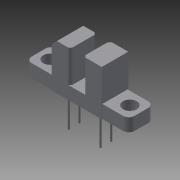
# Autodesk Inventor part: Capteur optique
Saved by Autodesk Inventor 2015 SP1 (Build 190203100, 203)
## iProperties
Created: 2015-05-01
Part Number: Capteur optique
Material: Générique
Document SubType Name: Modeling
Designer: Cyril
Density: 1 g/cm^3
Appearance: Par défaut
Author: Cyril
Autodesk Inventor part; units mm, degrees
ref_plane "YZ Plane" through (0, 0, 0) normal (1, 0, 0) x (0, 1, 0)
ref_plane "XZ Plane" through (0, 0, 0) normal (0, 1, 0) x (-1, 0, 0)
ref_plane "XY Plane" through (0, 0, 0) normal (0, 0, 1) x (1, 0, 0)
sketch "Sketch1" plane through (0, 0, 0) normal (0, 1, 0) x (-1, 0, 0)
  line L0 (-1.55, 2.6) -> (-5.95, 2.6)
  line L1 (-5.95, 2.6) -> (-5.95, -8.2)
  line L2 (-5.95, -8.2) -> (5.95, -8.2)
  line L3 (5.95, -8.2) -> (5.95, 1.4)
  line L4 (5.95, 1.4) -> (4.75, 2.6)
  line L5 (4.75, 2.6) -> (1.55, 2.6)
  line L6 (1.55, 2.6) -> (1.55, -5.1)
  line L7 (1.55, -5.1) -> (-1.55, -5.1)
  line L8 (-1.55, -5.1) -> (-1.55, 2.6)
  line L9 (0, -10.36) -> (0, 4.76) projected
  point P0 (0, 0)
  dimension "d0" = 11.9
  dimension "d1" = 10.8
  dimension "d2" = 2.6
  dimension "d3" = 3.1
  dimension "d4" = 3.1
  dimension "d5" = 135
  dimension "d6" = 1.2
  constraints: 18 end point, 6 perpendicular, 2 point on line, 1 horizontal, 2 other
  measures "d0" distance of L1.end L2.end
  measures "d1" distance of L0.end L1.end
  measures "d2" distance from line of point (0, 0) L0
  measures "d3" distance between parallel lines of L8 L6
  measures "d4" distance between parallel lines of L7 L2
  measures "d5" angle of L5 L4
  measures "d6" distance from line of L4.end L3
extrude "Extrusion1" add sketch "Sketch1" along normal mid plane 6.3
sketch "Sketch2" plane through (5.95, -3.15, -8.2) normal (1, 0, 0) x (0, 0, -1)
  line L0 (0, 0.15) -> (-3.1, 0.15)
  line L1 (-3.1, 0.15) -> (-3.1, 6.15)
  line L2 (-3.1, 6.15) -> (0, 6.15)
  line L3 (0, 6.15) -> (0, 0.15)
  line L4 (2.16, 3.15) -> (-12.96, 3.15) projected
  point P0 (-8.2, 3.15)
  point P1 (0, 0)
  dimension "d12" = 6
  dimension "d13" = 3.1
  constraints: 8 end point, 2 parallel, 1 horizontal, 1 perpendicular, 1 point on line, 1 other
  measures "d12" distance of L0.end L1.end
  measures "d13" distance of L1.end L2.end
extrude "Extrusion2" add sketch "Sketch2" along normal blind 6.3
fillet "Fillet1" radius 1.35 2 edges at (12.25, -3, -6.65) (12.25, 3, -6.65)
sketch "Sketch3" plane through (5.95, -3, -5.1) normal (0, 0, 1) x (1, 0, 0)
  circle A0 centre (3.55, 3) radius 1.65
  line L0 (0, -0.15) -> (0, 6.15) projected
  line L1 (-15.54, 3) -> (9.94, 3) projected
  point P0 (-5.95, 3)
  dimension "d15" = 3.3
  dimension "d16" = 3.55
  constraints: 1 centre point, 1 point on line
  measures "d15" diameter of A0
  measures "d16" distance from line of L0 A0.centre
extrude "Extrusion3" cut sketch "Sketch3" against normal through all
sketch "Sketch4" plane through (5.95, -3.15, -8.2) normal (0, 0, -1) x (-1, 0, 0)
  circle A0 centre (2.15, 1.88) radius 0.2
  circle A1 centre (2.15, 4.42) radius 0.2
  line L0 (5.95, -1.26) -> (5.95, 7.56) projected
  line L1 (2.15, 1.88) -> (2.15, 4.42) construction
  line L2 (-9.94, 3.15) -> (15.54, 3.15) projected
  point P0 (5.95, 3.15)
  dimension "d19" = 0.4
  dimension "d20" = 3.8
  dimension "d21" = 0.4
  dimension "d22" = 2.54
  constraints: 2 centre point, 2 end point, 1 symmetric about line, 1 vertical
  measures "d19" diameter of A0
  measures "d20" distance from line of L0 L1.start
  measures "d21" diameter of A1
  measures "d22" distance of L1.end L1.start
extrude "Extrusion4" add sketch "Sketch4" along normal blind 7.8
mirror "Mirror1" about plane through (0, 0, 0) normal (1, 0, 0) of "Extrusion2", "Fillet1", "Extrusion3", "Extrusion4"
chamfer "Chamfer1" distance 0.5 angle 45 4 edges at (1.55, 3.15, -1.25) (1.55, -3.15, -1.25) (-1.55, -3.15, -1.25) (-1.55, 3.15, -1.25)
equation "\"d21\" = d19"
body "Solid1"
